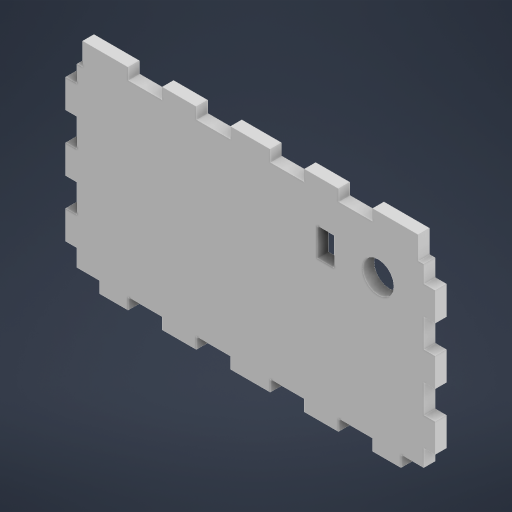
# Autodesk Inventor part: Langbektang houder
Saved by Autodesk Inventor 2023.2 (Build 272271000, 271)
## iProperties
Created: 2020-09-09
Part Number: Langbektang houder
Material: Generic
Document SubType Name: Modeling
Designer: nathan.bollaert
Density: 1 g/cm^3
Appearance: Default
Author: nathan.bollaert
Autodesk Inventor part; units mm, degrees
ref_plane "YZ Plane" through (0, 0, 0) normal (1, 0, 0) x (0, 1, 0)
ref_plane "XZ Plane" through (0, 0, 0) normal (0, 1, 0) x (-1, 0, 0)
ref_plane "XY Plane" through (0, 0, 0) normal (0, 0, 1) x (1, 0, 0)
sketch "Sketch1" plane through (0, 0, 0) normal (0, 0, 1) x (1, 0, 0)
  line L0 (0, -74) -> (130, -74)
  line L1 (130, -74) -> (130, 0)
  line L2 (130, 0) -> (0, 0)
  line L3 (0, 0) -> (0, -74)
  dimension "d228" = 130
  dimension "d229" = 74
  constraints: 8 end point, 2 parallel, 1 coincident, 1 horizontal, 1 perpendicular
  measures "d228" distance of L2.end L1.end
  measures "d229" distance of L1.end L0.end
extrude "Extrusion1" add sketch "Sketch1" against normal blind 4
sketch "Sketch2" plane through (0, 0, 0) normal (0, 0, 1) x (1, 0, 0)
  line L0 (0, -74) -> (0, 0) projected
  line L1 (0, -37) -> (130, -37)
  line L2 (130, 0) -> (130, -74) projected
  line L3 (65, 0) -> (65, -74)
  line L4 (130, -74) -> (0, -74) projected
  line L5 (22, -74) -> (12, -74)
  line L6 (12, -74) -> (12, -70)
  line L7 (22, -70) -> (22, -74)
  line L8 (46, -70) -> (46, -74)
  line L9 (46, -74) -> (34, -74)
  line L10 (34, -74) -> (34, -70)
  line L11 (72, -70) -> (72, -74)
  line L12 (72, -74) -> (58, -74)
  line L13 (58, -74) -> (58, -70)
  line L14 (0, -74) -> (130, -74) projected
  line L15 (96, -74) -> (84, -74)
  line L16 (84, -74) -> (84, -70)
  line L17 (96, -70) -> (96, -74)
  line L18 (118, -70) -> (118, -74)
  line L19 (118, -74) -> (108, -74)
  line L20 (108, -74) -> (108, -70)
  line L21 (0, -54) -> (4, -54)
  line L22 (4, -54) -> (4, -44)
  line L23 (4, -44) -> (0, -44)
  line L24 (0, -44) -> (0, -54)
  line L25 (0, -34) -> (4, -34)
  line L26 (4, -34) -> (4, -24)
  line L27 (4, -24) -> (0, -24)
  line L28 (0, -24) -> (0, -34)
  line L29 (0, 0) -> (0, -74) projected
  line L30 (130, -74) -> (130, 0)
  line L31 (130, 0) -> (130, -74)
  line L32 (0, -70) -> (12, -70)
  line L33 (22, -70) -> (34, -70)
  line L34 (46, -70) -> (58, -70)
  line L35 (72, -70) -> (84, -70)
  line L36 (96, -70) -> (108, -70)
  line L37 (118, -70) -> (130, -70)
  line L38 (0, 0) -> (0, -74)
  line L39 (6, 0) -> (6, -8)
  line L40 (22, -4) -> (22, 0)
  line L41 (46, -4) -> (46, 0)
  line L42 (46, 0) -> (34, 0)
  line L43 (34, 0) -> (34, -4)
  line L44 (72, -4) -> (72, 0)
  line L45 (72, 0) -> (58, 0)
  line L46 (58, 0) -> (58, -4)
  line L47 (96, -4) -> (96, 0)
  line L48 (108, 0) -> (108, -4)
  line L49 (96, 0) -> (84, 0)
  line L50 (84, 0) -> (84, -4)
  line L51 (0, -74) -> (0, 0)
  line L52 (130, 0) -> (130, -74)
  line L53 (130, -74) -> (130, 0)
  line L54 (22, -4) -> (34, -4)
  line L55 (46, -4) -> (58, -4)
  line L56 (72, -4) -> (84, -4)
  line L57 (96, -4) -> (108, -4)
  line L58 (130, -74) -> (130, 0)
  line L59 (130, 0) -> (130, -74)
  line L60 (130, 0) -> (130, -74)
  line L61 (130, -74) -> (130, 0)
  line L62 (0, -70) -> (4, -70)
  line L63 (4, -70) -> (4, -64)
  line L64 (4, -64) -> (0, -64)
  line L65 (0, -64) -> (0, -70)
  line L66 (0, -4) -> (4, -4)
  line L67 (4, -4) -> (4, -14)
  line L68 (4, -14) -> (0, -14)
  line L69 (0, -14) -> (0, -4)
  line L70 (130, -74) -> (130, 0)
  line L71 (130, -54) -> (126, -54)
  line L72 (126, -54) -> (126, -44)
  line L73 (126, -44) -> (130, -44)
  line L74 (130, -44) -> (130, -54)
  line L75 (126, -34) -> (126, -24)
  line L76 (130, -34) -> (126, -34)
  line L77 (126, -24) -> (130, -24)
  line L78 (130, -24) -> (130, -34)
  line L79 (130, 0) -> (130, -74)
  line L80 (130, 0) -> (130, -74)
  line L81 (130, -74) -> (130, 0)
  line L82 (130, -70) -> (126, -70)
  line L83 (126, -70) -> (126, -64)
  line L84 (126, -64) -> (130, -64)
  line L85 (130, -64) -> (130, -70)
  line L86 (130, -4) -> (126, -4)
  line L87 (126, -4) -> (126, -14)
  line L88 (126, -14) -> (130, -14)
  line L89 (130, -14) -> (130, -4)
  line L90 (130, 0) -> (0, 0) projected
  line L91 (6, -8) -> (0, -8)
  line L92 (124, 0) -> (124, -8)
  line L93 (124, -8) -> (130, -8)
  point P0 (58, -74)
  point P1 (72, -74)
  point P2 (0, -24)
  point P3 (0, -34)
  point P4 (84, -74)
  point P5 (96, -74)
  point P6 (0, -44)
  point P7 (130, -70)
  point P8 (0, -70)
  point P9 (0, -14)
  point P10 (0, -64)
  point P11 (126, -70)
  point P12 (130, -64)
  point P13 (130, -54)
  point P14 (130, -44)
  point P15 (130, -34)
  point P16 (130, -14)
  point P17 (0, -8)
  point P18 (126, -8)
  dimension "d234" = 10
  dimension "d235" = 12
  dimension "d236" = 12
  dimension "d237" = 12
  dimension "d238" = 14
  dimension "d240" = 12
  dimension "d242" = 12
  dimension "d243" = 10
  dimension "d244" = 12
  dimension "d245" = 12
  dimension "d246" = 12
  dimension "d249" = 10
  dimension "d251" = 10
  dimension "d255" = 10
  dimension "d262" = 4
  dimension "d267" = 10
  dimension "d268" = 10
  dimension "d271" = 10
  dimension "d272" = 14
  dimension "d274" = 6
  dimension "d278" = 8
  constraints: 176 end point, 44 symmetric about line, 31 equal length, 16 point on line, 8 perpendicular, 7 horizontal, 3 midpoint, 1 vertical, 1 vertical alignment, 9 other
  measures "d234" distance between parallel lines of L7 L6
  measures "d235" distance between parallel lines of L0 L6
  measures "d236" distance of L8.end L9.end
  measures "d237" distance between parallel lines of L10 L7
  measures "d238" distance of L11.end L12.end
  measures "d240" distance of L8.end L12.end
  measures "d242" distance between parallel lines of L17 L16
  measures "d243" distance of L18.end L19.end
  measures "d244" distance between parallel lines of L20 L17
  measures "d245" distance of L11.end L15.end
  measures "d246" distance of L2.end L18.end
  measures "d249" distance between parallel lines of L23 L21
  measures "d251" distance between parallel lines of L27 L25
  measures "d255" distance between parallel lines of L23 L25
  measures "d262" distance between parallel lines of L4 L32
  measures "d267" distance of L38.end L64.end
  measures "d268" distance of L21.start L64.end
  measures "d271" distance of L27.end L68.end
  measures "d272" distance of L0.end L68.end
  measures "d274" distance between parallel lines of L38 L39
  measures "d278" distance of the line from the sketch origin of L91
extrude "Extrusion2" cut sketch "Sketch2" against normal blind 4 contours L0 L32 L6 L4 | L0 L64 L63 L32 | L7 L33 L10 L4 | L0 L23 L22 L21 | L8 L34 L13 L4 | L0 L27 L26 L25 | L11 L35 L16 L4 | L0 L91 L67 L68 | L76 L75 L77 L2 | L2 L71 L72 L73 | L90 L50 L56 L44 | L46 L55 L41 L90 | L0 L66 L67 L91 | L17 L36 L20 L4 | L0 L90 L39 L91 L67 L66 | L88 L87 L93 L2 | L2 L37 L83 L84 | L90 L48 L57 L47 | L43 L54 L40 L90 | L93 L87 L86 L2 | L2 L4 L18 L37 | L86 L87 L93 L92 L90 L2
sketch "Sketch3" plane through (0, 0, -4) normal (0, 0, -1) x (-1, 0, 0)
  circle A0 centre (-110, -20) radius 5.5
  line L0 (-130, -14) -> (-130, -24) projected
  line L1 (-108, 0) -> (-124, 0) projected
  point P0 (0, 0)
  dimension "d279" = 11
  dimension "d280" = 20
  dimension "d281" = 20
  constraints: 1 centre point
  measures "d279" diameter of A0
  measures "d280" distance from line of L0 A0.centre
  measures "d281" distance from line of L1 A0.centre
extrude "Extrusion3" cut sketch "Sketch3" against normal blind 4
sketch "Sketch4" plane through (0, 0, -4) normal (0, 0, -1) x (-1, 0, 0)
  line L0 (-94.5, -15) -> (-88.5, -15)
  line L1 (-88.5, -15) -> (-88.5, -25)
  line L2 (-88.5, -25) -> (-94.5, -25)
  line L3 (-94.5, -25) -> (-94.5, -15)
  circle A0 centre (-110, -20) radius 5.5 projected
  point P0 (0, 0)
  point P1 (-94.5, -20)
  dimension "d297" = 10
  dimension "d298" = 10
  dimension "d299" = 6
  constraints: 8 end point, 2 parallel, 1 horizontal, 1 horizontal alignment, 1 midpoint, 1 perpendicular
  measures "d297" distance of L0.end L1.end
  measures "d298" distance edge to line of A0 L3
  measures "d299" distance of L0.start L0.end
extrude "Extrusion4" cut sketch "Sketch4" against normal blind 4 contours L0 L1 L2 L3
body "Solid5"
